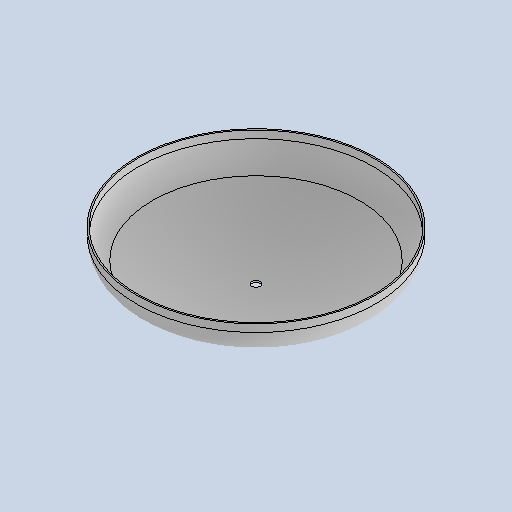
# Autodesk Inventor part: PNS - 604 dished head D1000
Saved by Autodesk Inventor 2025 (Build 290162010, 162A)
## iProperties
Created: 2025-02-16
Part Number: PNS - 604 dished head D1000
Material: Generic
Document SubType Name: Modeling
Designer: pokla
Density: 1 g/cm^3
Appearance: Default
Disherd_head_hight: 205.000 mm
Author: pokla
Autodesk Inventor part; units mm, degrees
ref_plane "YZ Plane" through (0, 0, 0) normal (1, 0, 0) x (0, 1, 0)
ref_plane "XZ Plane" through (0, 0, 0) normal (0, 1, 0) x (-1, 0, 0)
ref_plane "XY Plane" through (0, 0, 0) normal (0, 0, 1) x (1, 0, 0)
sketch "Sketch1" plane through (0, 0, 0) normal (0, 1, 0) x (-1, 0, 0)
  line L0 (476, 0) -> (476, -30)
  arc A0 (414.3671, -122.347) -> (476, -30) centre (376, -30) ccw
  arc A1 (0, -205) -> (414.3671, -122.347) centre (0, 875.0067) ccw
  line L1 (0, 191.6842) -> (0, -191.6842)
  arc A2 (0, -199) -> (412.0651, -116.8062) centre (0, 875.0067) ccw
  arc A3 (412.0651, -116.8062) -> (470, -30) centre (376, -30) ccw
  line L2 (470, -30) -> (470, 0)
  line L3 (470, 0) -> (476, 0)
  line L4 (0, -199) -> (0, -205)
  point P0 (0, 0)
  point P1 (0, 0)
  point P2 (0, -202)
  point P3 (0, -163.7009)
  point P4 (0, -169.7009)
  dimension "d0" = 100
  dimension "d1" = 30
  dimension "d3" = 1080.0067
  dimension "d6" = 6
  dimension "d11" = 940
  dimension "d12" = 205
  constraints: 10 end point, 8 point on circle, 4 centre point, 2 midpoint, 2 tangent, 2 vertical, 1 coincident, 1 horizontal, 1 horizontal alignment, 1 line through centre, 1 parallel, 1 vertical alignment, 2 other
  measures "d0" radius of A0
  measures "d1" distance of L0.start L0.end
  measures "d3" radius of A1
  measures "d6" radial gap between concentric circles of A1 A2
  measures "d11" diameter of L2 L1
  measures "d12" distance of L4.end point (0, 0)
revolve "Revolution1" add sketch "Sketch1" angle 360 about axis through (0, 0, 191.6842) along (0, 0, -1)
sketch "Sketch2" plane through (0, 0, 0) normal (0, 0, 1) x (1, 0, 0)
  circle A0 centre (0, 0) radius 16.75
  dimension "d8" = 33.5
  constraints: 1 centre point, 1 coincident
  measures "d8" diameter of A0
extrude "Extrusion1" cut sketch "Sketch2" against normal through all
equation "\"d11\" = MAIN_filter_diam"
equation "\"Disherd_head_hight\" = d12"
equation "\"MAIN_filter_diam\" = 940"
body "Solid1"
